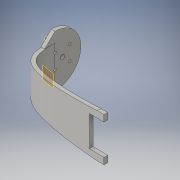
# Autodesk Inventor part: backplaterev2.0
Saved by Autodesk Inventor 2016 (Build 200138000, 138)
## iProperties
Created: 2017-03-21
Part Number: backplaterev2.0
Material: Generic
Document SubType Name: Modeling
Designer: Jorian Bruslind
Density: 1 g/cm^3
Appearance: Default
Author: Jorian Bruslind
Autodesk Inventor part; units mm, degrees
ref_plane "YZ Plane" through (0, 0, 0) normal (1, 0, 0) x (0, 1, 0)
ref_plane "XZ Plane" through (0, 0, 0) normal (0, 1, 0) x (-1, 0, 0)
ref_plane "XY Plane" through (0, 0, 0) normal (0, 0, 1) x (1, 0, 0)
sketch "Sketch5" plane through (0, 0, 0) normal (0, 1, 0) x (-1, 0, 0)
  line L0 (0, 0) -> (82.55, 0) construction
  line L1 (82.55, 0) -> (154.5063, -11.1125) construction
  line L2 (154.5063, -11.1125) -> (165.1, -20.751) construction
  line L3 (165.1, -20.751) -> (165.1, -74.6252) construction
  spline S0 degree 4 poles (0, 0) (82.55, 0) (154.5063, -11.1125) (165.1, -20.751) (165.1, -74.6252) knots 1 1 1 1 1 2 2 2 2 2
  line L4 (165.1, -74.6252) -> (158.7373, -74.6252)
  line L5 (0, 0) -> (0, -6.3627)
  spline S1 degree 5 poles (0, -6.3627) (7.0757, -6.3627) (14.1514, -6.4398) (21.2259, -6.5911) (34.7743, -7.0225) (48.3104, -7.7412) (54.7765, -8.1539) (66.8772, -9.0681) (78.9498, -10.2962) (84.5682, -10.9466) (94.8197, -12.3033) (105.0089, -14.0632) (109.6069, -14.9605) (117.7528, -16.7786) (125.7539, -19.1506) (129.2212, -20.3232) (135.2073, -22.6734) (140.8452, -25.7516) (143.1816, -27.234) (147.282, -30.3883) (150.6692, -34.2889) (152.0422, -36.2659) (154.5965, -40.9141) (156.218, -45.974) (156.8738, -48.8034) (158.0603, -55.6306) (158.5355, -62.5498) (158.6819, -66.5724) (158.737, -70.5995) (158.7373, -74.6252) knots 0 0 0 0 0 0 0.178602 0.178602 0.178602 0.342136 0.342136 0.342136 0.484884 0.484884 0.484884 0.603095 0.603095 0.603095 0.69542 0.69542 0.69542 0.765007 0.765007 0.765007 0.82525 0.82525 0.82525 0.898378 0.898378 0.898378 1 1 1 1 1 1
  dimension "d24" = 6.3627
  constraints: 4 end point, 1 horizontal, 1 perpendicular, 6 other
extrude "Extrusion4" add sketch "Sketch5" along normal blind 76.2
ref_plane "Work Plane2" through (-103.6581, 76.2, -7.4114) normal (-0.1753747, 0, 0.9845018) x (0, -1, 0)
sketch "Sketch7" plane through (-103.6581, 76.2, -7.4114) normal (-0.1753747, 0, 0.9845018) x (0, -1, 0)
  line L0 (76.2, 103.3513) -> (63.5, 103.3513)
  line L1 (76.2, 103.3513) -> (0, 103.3513) projected
  line L2 (63.5, 103.3513) -> (63.5, -87.1487)
  line L3 (63.5, -87.1487) -> (12.7, -87.1487)
  line L4 (63.5, -87.1487) -> (76.2, 103.3513)
  line L5 (12.7, -87.1487) -> (0, 103.3513)
  line L6 (76.2, 103.3513) -> (0, 103.3513)
  line L7 (0, 103.3513) -> (0, -87.1487)
  line L8 (0, -87.1487) -> (76.2, -87.1487)
  line L9 (76.2, -87.1487) -> (76.2, 103.3513)
  dimension "d27" = 12.7
  dimension "d28" = 190.5
  dimension "d29" = 50.8
  constraints: 18 end point, 2 horizontal, 2 parallel, 2 perpendicular, 1 point on line
  measures "d27" distance of L0.start L0.end
  measures "d28" distance of L0.end L2.end
  measures "d29" distance of L2.end L3.end
extrude "Extrusion5" cut sketch "Sketch7" against normal blind 76.2 contours L9 L8 L4 | L5 L8 L7
ref_plane "Work Plane3" through (-165.1, 64.4914, -74.6252) normal (-1, 0, 0) x (0, -1, 0)
sketch "Sketch8" plane through (-165.1, 64.4914, -74.6252) normal (-1, 0, 0) x (0, -1, 0)
  line L0 (52.7829, 0) -> (0, 0) projected
  line L1 (0, 0) -> (26.3914, 0)
  circle A0 centre (26.3914, 0) radius 44.45
  line L2 (-18.0586, 0) -> (0, 18.0586)
  line L3 (52.7829, 18.0586) -> (70.8414, 0)
  line L4 (0, 18.0586) -> (52.7829, 18.0586)
  point P0 (64.4914, 74.6252)
  dimension "d32" = 88.9
  constraints: 8 end point, 2 point on circle, 1 centre point, 1 coincident, 1 horizontal, 1 midpoint, 1 perpendicular
  measures "d32" diameter of A0
extrude "Extrusion6" add sketch "Sketch8" against normal blind 6.3627 contours A0 L2 L4 L3 picked at (27.9402, -2.6964)
sketch "Sketch10" plane through (0, 0, 0) normal (1, 0, 0) x (0, 0, -1)
  line L0 (0, 0) -> (0, 0.7937)
  line L1 (0, 0) -> (0, 76.2) projected
  line L2 (0, 76.2) -> (0, 75.4126)
  line L3 (0, 75.4126) -> (0, 64.2874)
  line L4 (0, 0.7937) -> (0, 11.9189)
  line L5 (0, 11.9189) -> (7.62, 11.9189)
  line L6 (7.62, 11.9189) -> (7.62, 64.2874)
  line L7 (7.62, 64.2874) -> (0, 64.2874)
  line L8 (0, 64.2874) -> (0, 11.9189)
  line L9 (0, 76.2) -> (7.62, 76.2)
  line L10 (7.62, 76.2) -> (7.62, 75.4126)
  line L11 (7.62, 75.4126) -> (0, 75.4126)
  line L12 (0, 75.4126) -> (0, 76.2)
  line L13 (0, 0.7937) -> (7.62, 0.7937)
  line L14 (7.62, 0.7937) -> (7.62, 0.0064)
  line L15 (7.62, 0.0064) -> (0, 0.0064)
  line L16 (0, 0.0064) -> (0, 0.7937)
  dimension "d47" = 0.7937
  dimension "d48" = 0.7874
  dimension "d49" = 11.1252
  dimension "d50" = 11.1252
  dimension "d51" = 7.62
  dimension "d52" = 7.62
  dimension "d53" = 7.62
  dimension "d54" = 0.7874
  constraints: 32 end point, 6 parallel, 4 point on line, 3 horizontal, 3 perpendicular
  measures "d47" distance of L0.start L0.end
  measures "d48" distance of L1.end L2.end
  measures "d49" distance of L2.end L3.end
  measures "d50" distance of L0.end L4.end
  measures "d51" distance of L7.end L6.end
  measures "d52" distance of L10.end L11.end
  measures "d53" distance of L14.end L15.end
  measures "d54" distance of L13.end L14.end
extrude "Extrusion8" cut sketch "Sketch10" against normal blind 25.4
sketch "Sketch11" plane through (-165.1, 64.4914, -74.6252) normal (-1, 0, 0) x (0, 0, 1)
  arc A0 (0, 18.0586) -> (0, -70.8414) centre (0, -26.3914) ccw projected
  line L0 (0, -70.8414) -> (0, 18.0586)
  line L1 (0, -53.2005) -> (0, 0.4176) projected
  line L2 (0, -26.3914) -> (-12.7, -26.3914)
  line L3 (-12.7, -26.3914) -> (-25.4, -26.3914)
  line L4 (-25.4, -26.3914) -> (-25.4, -13.6914)
  line L5 (-25.4, -26.3914) -> (-25.4, -39.0914)
  line L6 (0, -26.3914) -> (0, -13.6914)
  line L7 (0, -26.3914) -> (0, -39.0914)
  circle A1 centre (0, -39.0914) radius 2
  circle A2 centre (0, -13.6914) radius 2
  circle A3 centre (-25.4, -13.6914) radius 2
  circle A4 centre (-25.4, -39.0914) radius 2
  circle A5 centre (-12.7, -26.3914) radius 3.81
  point P0 (74.6252, -64.4914)
  dimension "d57" = 12.7
  dimension "d58" = 12.7
  dimension "d59" = 12.7
  dimension "d60" = 12.7
  dimension "d61" = 12.7
  dimension "d62" = 12.7
  dimension "d63" = 4
  dimension "d64" = 4
  dimension "d65" = 4
  dimension "d66" = 4
  dimension "d69" = 7.62
  constraints: 14 end point, 5 centre point, 5 coincident, 3 point on line, 1 collinear, 1 horizontal, 1 perpendicular, 1 vertical
  measures "d57" distance of L2.start L2.end
  measures "d58" distance of L2.end L3.end
  measures "d59" distance of L3.end L4.end
  measures "d60" distance of L3.end L5.end
  measures "d61" distance of L2.start L6.end
  measures "d62" distance of L2.start L7.end
  measures "d63" diameter of A1
  measures "d64" diameter of A2
  measures "d65" diameter of A3
  measures "d66" diameter of A4
  measures "d69" diameter of A5
extrude "Extrusion10" cut sketch "Sketch11" against normal blind 7.62 contours A2 L0 | L0 A2 | A1 L0 | L0 A1 | A5 L3 L2 | L2 L3 A5 | A3 | A4
sketch "Sketch12" plane through (-165.1, 64.4914, -74.6252) normal (-1, 0, 0) x (0, -1, 0)
  line L0 (11.6914, 0) -> (-0.4176, 0) projected
  line L1 (-0.4176, 0) -> (-0.4176, -12.7)
  circle A0 centre (-0.4176, -12.7) radius 3.5
  circle A1 centre (-0.4176, -12.7) radius 4.5
  point P0 (64.4914, 74.6252)
  dimension "d72" = 12.7
  dimension "d73" = 7
  dimension "d74" = 9
  constraints: 2 centre point, 2 coincident, 2 end point, 1 vertical
  measures "d72" distance of L0.end L1.end
  measures "d73" diameter of A0
  measures "d74" diameter of A1
extrude "Extrusion11" add sketch "Sketch12" along normal blind 2
sketch "Sketch13" plane through (-167.1, 64.909, -87.3252) normal (-1, 0, 0) x (0, 0, 1)
  line L0 (0, 0) -> (0, 5.08)
  line L1 (0, 5.08) -> (-0.635, 5.08)
  line L2 (-0.635, 5.08) -> (0.635, 5.08)
  line L3 (0.635, 5.08) -> (0.635, -5.08)
  line L4 (0.635, -5.08) -> (-0.635, -5.08)
  line L5 (-0.635, -5.08) -> (-0.635, 5.08)
  point P0 (87.3252, -64.909)
  dimension "d82" = 5.08
  dimension "d83" = 0.635
  dimension "d84" = 1.27
  dimension "d85" = 10.16
  constraints: 12 end point, 2 parallel, 2 perpendicular, 1 horizontal, 1 vertical
  measures "d82" distance of L0.start L0.end
  measures "d83" distance of L0.end L1.end
  measures "d84" distance of L3.end L4.end
  measures "d85" distance of L2.end L3.end
extrude "Extrusion12" cut sketch "Sketch13" against normal blind 2
body "Solid3"
